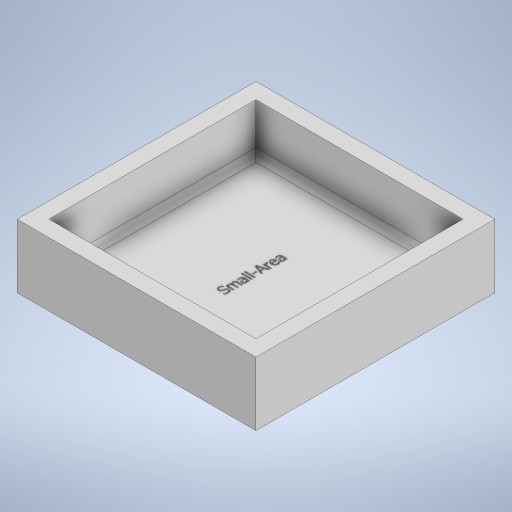
# Autodesk Inventor part: Small_Tower
Saved by Autodesk Inventor 2024.3 (Build 283343000, 343)
## iProperties
Created: 2024-08-06
Part Number: Small_Tower
Material: Generic
Document SubType Name: Modeling
Designer: lordk
Density: 1 g/cm^3
Appearance: Default
Author: lordk
Autodesk Inventor part; units mm, degrees
ref_plane "YZ Plane" through (0, 0, 0) normal (1, 0, 0) x (0, 1, 0)
ref_plane "XZ Plane" through (0, 0, 0) normal (0, 1, 0) x (-1, 0, 0)
ref_plane "XY Plane" through (0, 0, 0) normal (0, 0, 1) x (1, 0, 0)
sketch "Sketch1" plane through (0, 0, 0) normal (0, 1, 0) x (-1, 0, 0)
  line L0 (-37.5, 37.5) -> (37.5, 37.5)
  line L1 (37.5, 37.5) -> (37.5, -37.5)
  line L2 (37.5, -37.5) -> (-37.5, -37.5)
  line L3 (-37.5, -37.5) -> (-37.5, 37.5)
  line L4 (-37.5, 37.5) -> (37.5, -37.5) construction
  line L5 (37.5, 37.5) -> (-37.5, -37.5) construction
  point P0 (0, 0)
  dimension "d0" = 75
  dimension "d1" = 75
  constraints: 12 end point, 2 midpoint, 2 parallel, 1 horizontal, 1 perpendicular
  measures "d0" distance of L1.end L2.end
  measures "d1" distance of L0.end L1.end
extrude "Extrusion1" add sketch "Sketch1" along normal blind 20
sketch "Sketch2" plane through (0, 20, 0) normal (0, 1, 0) x (1, 0, 0)
  point P0 (0, 0)
shell "Shell1" thickness 5 removed faces 1 at (12.5, 20, 12.5)
fillet "Fillet1" radius 2 4 edges at (-32.5, 5, 0) (0, 5, -32.5) (0, 5, 32.5) (32.5, 5, 0)
sketch "Sketch3" plane through (-30.5, 5, -30.5) normal (0, 1, 0) x (1, 0, 0)
  line L0 (28, -41) -> (28, -20) construction
  line L1 (28, -20) -> (31, -20) construction
  line L2 (31, -20) -> (31, -41) construction
  line L3 (31, -41) -> (28, -41) construction
  line L4 (-2, 2) -> (-2, -63) projected
  line L5 (0, 0) -> (61, 0) projected
  line L6 (61, -61) -> (0, -61) projected
  line L7 (61, 0) -> (61, -61) projected
  spline S0 degree 2 poles (31.2382, -39.8416) (31.2382, -40.1725) (31.0999, -40.6369) (31.0011, -40.8419) knots 0 0 0 1 2 2 2
  line L8 (31.0011, -40.8419) -> (30.4922, -40.8419)
  line L9 (30.4922, -40.8419) -> (30.4922, -40.8123)
  spline S1 degree 2 poles (30.4922, -40.8123) (30.68, -40.6122) (30.8874, -40.1059) (30.8874, -39.8712) knots 0 0 0 1 2 2 2
  spline S2 degree 2 poles (30.8874, -39.8712) (30.8874, -39.5353) (30.6083, -39.1919) (30.3786, -39.1919) knots 0 0 0 1 2 2 2
  spline S3 degree 2 poles (30.3786, -39.1919) (30.1958, -39.1919) (29.9686, -39.3723) (29.9118, -39.5674) knots 0 0 0 1 2 2 2
  spline S4 degree 2 poles (29.9118, -39.5674) (29.8723, -39.7082) (29.8179, -39.9428) (29.7735, -40.1182) knots 0 0 0 1 2 2 2
  spline S5 degree 2 poles (29.7735, -40.1182) (29.7315, -40.2763) (29.6055, -40.5258) (29.5042, -40.6221) knots 0 0 0 1 2 2 2
  spline S6 degree 2 poles (29.5042, -40.6221) (29.403, -40.7159) (29.1313, -40.8197) (28.9534, -40.8197) knots 0 0 0 1 2 2 2
  spline S7 degree 2 poles (28.9534, -40.8197) (28.5829, -40.8197) (28.0815, -40.2417) (28.0815, -39.7946) knots 0 0 0 1 2 2 2
  spline S8 degree 2 poles (28.0815, -39.7946) (28.0815, -39.5378) (28.1828, -39.0833) (28.2791, -38.8881) knots 0 0 0 1 2 2 2
  line L10 (28.2791, -38.8881) -> (28.7632, -38.8881)
  line L11 (28.7632, -38.8881) -> (28.7632, -38.9178)
  spline S9 degree 2 poles (28.7632, -38.9178) (28.6299, -39.0635) (28.4323, -39.518) (28.4323, -39.7675) knots 0 0 0 1 2 2 2
  spline S10 degree 2 poles (28.4323, -39.7675) (28.4323, -40.049) (28.6965, -40.3973) (28.9114, -40.3973) knots 0 0 0 1 2 2 2
  spline S11 degree 2 poles (28.9114, -40.3973) (29.1041, -40.3973) (29.3338, -40.1923) (29.3857, -39.9996) knots 0 0 0 1 2 2 2
  spline S12 degree 2 poles (29.3857, -39.9996) (29.4203, -39.8712) (29.5092, -39.4982) (29.5462, -39.3747) knots 0 0 0 1 2 2 2
  spline S13 degree 2 poles (29.5462, -39.3747) (29.6426, -39.061) (30.0304, -38.7696) (30.3144, -38.7696) knots 0 0 0 1 2 2 2
  spline S14 degree 2 poles (30.3144, -38.7696) (30.4947, -38.7696) (30.8405, -38.9153) (30.9615, -39.0462) knots 0 0 0 1 2 2 2
  spline S15 degree 2 poles (30.9615, -39.0462) (31.0949, -39.1919) (31.2382, -39.5625) (31.2382, -39.8416) knots 0 0 0 1 2 2 2
  line L12 (31.1839, -35.7932) -> (29.8599, -35.7932)
  spline S16 degree 2 poles (29.8599, -35.7932) (29.7018, -35.7932) (29.4326, -35.8179) (29.3585, -35.8574) knots 0 0 0 1 2 2 2
  spline S17 degree 2 poles (29.3585, -35.8574) (29.277, -35.8969) (29.198, -36.0476) (29.198, -36.1785) knots 0 0 0 1 2 2 2
  spline S18 degree 2 poles (29.198, -36.1785) (29.198, -36.2971) (29.3437, -36.5688) (29.482, -36.7121) knots 0 0 0 1 2 2 2
  spline S19 degree 2 poles (29.482, -36.7121) (29.5166, -36.7096) (29.6129, -36.7046) (29.6771, -36.7046) knots 0 0 0 1 2 2 2
  line L13 (29.6771, -36.7046) -> (31.1839, -36.7046)
  line L14 (31.1839, -36.7046) -> (31.1839, -37.09)
  line L15 (31.1839, -37.09) -> (29.8599, -37.09)
  spline S20 degree 2 poles (29.8599, -37.09) (29.7018, -37.09) (29.4326, -37.1147) (29.3585, -37.1542) knots 0 0 0 1 2 2 2
  spline S21 degree 2 poles (29.3585, -37.1542) (29.277, -37.1937) (29.198, -37.3444) (29.198, -37.4753) knots 0 0 0 1 2 2 2
  spline S22 degree 2 poles (29.198, -37.4753) (29.198, -37.5988) (29.3536, -37.873) (29.4746, -38.0014) knots 0 0 0 1 2 2 2
  line L16 (29.4746, -38.0014) -> (31.1839, -38.0014)
  line L17 (31.1839, -38.0014) -> (31.1839, -38.3867)
  line L18 (31.1839, -38.3867) -> (28.8966, -38.3867)
  line L19 (28.8966, -38.3867) -> (28.8966, -38.0014)
  line L20 (28.8966, -38.0014) -> (29.1486, -38.0014)
  spline S23 degree 2 poles (29.1486, -38.0014) (28.9979, -37.8507) (28.8324, -37.5543) (28.8324, -37.3765) knots 0 0 0 1 2 2 2
  spline S24 degree 2 poles (28.8324, -37.3765) (28.8324, -37.1739) (29.0176, -36.8603) (29.2276, -36.7787) knots 0 0 0 1 2 2 2
  spline S25 degree 2 poles (29.2276, -36.7787) (29.0325, -36.6034) (28.8324, -36.2724) (28.8324, -36.0797) knots 0 0 0 1 2 2 2
  spline S26 degree 2 poles (28.8324, -36.0797) (28.8324, -35.9315) (28.9238, -35.6895) (29.0275, -35.6005) knots 0 0 0 1 2 2 2
  spline S27 degree 2 poles (29.0275, -35.6005) (29.1313, -35.5092) (29.4425, -35.4079) (29.6771, -35.4079) knots 0 0 0 1 2 2 2
  line L21 (29.6771, -35.4079) -> (31.1839, -35.4079)
  line L22 (31.1839, -35.4079) -> (31.1839, -35.7932)
  spline S28 degree 2 poles (30.9418, -33.5924) (30.9764, -33.6394) (31.0999, -33.7974) (31.1369, -33.8715) knots 0 0 0 1 2 2 2
  spline S29 degree 2 poles (31.1369, -33.8715) (31.1913, -33.9728) (31.2481, -34.163) (31.2481, -34.3359) knots 0 0 0 1 2 2 2
  spline S30 degree 2 poles (31.2481, -34.3359) (31.2481, -34.4767) (31.1419, -34.7311) (31.0455, -34.8274) knots 0 0 0 1 2 2 2
  spline S31 degree 2 poles (31.0455, -34.8274) (30.9517, -34.9188) (30.675, -35.03) (30.5219, -35.03) knots 0 0 0 1 2 2 2
  spline S32 degree 2 poles (30.5219, -35.03) (30.2848, -35.03) (29.9488, -34.8299) (29.8525, -34.6125) knots 0 0 0 1 2 2 2
  spline S33 degree 2 poles (29.8525, -34.6125) (29.7636, -34.4199) (29.6969, -33.8962) (29.6796, -33.5924) knots 0 0 0 1 2 2 2
  line L23 (29.6796, -33.5924) -> (29.6055, -33.5924)
  spline S34 degree 2 poles (29.6055, -33.5924) (29.4721, -33.5924) (29.3066, -33.6739) (29.2597, -33.748) knots 0 0 0 1 2 2 2
  spline S35 degree 2 poles (29.2597, -33.748) (29.2128, -33.8221) (29.1831, -34.0346) (29.1831, -34.1482) knots 0 0 0 1 2 2 2
  spline S36 degree 2 poles (29.1831, -34.1482) (29.1831, -34.2816) (29.2622, -34.6422) (29.3387, -34.8225) knots 0 0 0 1 2 2 2
  line L24 (29.3387, -34.8225) -> (29.3387, -34.8447)
  line L25 (29.3387, -34.8447) -> (28.946, -34.8447)
  spline S37 degree 2 poles (28.946, -34.8447) (28.9164, -34.7385) (28.8423, -34.3408) (28.8423, -34.1457) knots 0 0 0 1 2 2 2
  spline S38 degree 2 poles (28.8423, -34.1457) (28.8423, -33.9086) (28.9164, -33.585) (29.0127, -33.4566) knots 0 0 0 1 2 2 2
  spline S39 degree 2 poles (29.0127, -33.4566) (29.1066, -33.3306) (29.4054, -33.2071) (29.6203, -33.2071) knots 0 0 0 1 2 2 2
  line L26 (29.6203, -33.2071) -> (31.1839, -33.2071)
  line L27 (31.1839, -33.2071) -> (31.1839, -33.5924)
  line L28 (31.1839, -33.5924) -> (30.9418, -33.5924)
  line L29 (30.6207, -33.5924) -> (29.9859, -33.5924)
  spline S40 degree 2 poles (29.9859, -33.5924) (29.9982, -33.7307) (30.0402, -34.1482) (30.0798, -34.2791) knots 0 0 0 1 2 2 2
  spline S41 degree 2 poles (30.0798, -34.2791) (30.1267, -34.4322) (30.3218, -34.6323) (30.4947, -34.6323) knots 0 0 0 1 2 2 2
  spline S42 degree 2 poles (30.4947, -34.6323) (30.6923, -34.6323) (30.8924, -34.41) (30.8924, -34.1976) knots 0 0 0 1 2 2 2
  spline S43 degree 2 poles (30.8924, -34.1976) (30.8924, -34.0173) (30.7368, -33.7209) (30.6207, -33.5924) knots 0 0 0 1 2 2 2
  line L30 (31.1839, -32.2734) -> (31.1839, -32.6588)
  line L31 (31.1839, -32.6588) -> (28, -32.6588)
  line L32 (28, -32.6588) -> (28, -32.2734)
  line L33 (28, -32.2734) -> (31.1839, -32.2734)
  line L34 (31.1839, -31.3151) -> (31.1839, -31.7004)
  line L35 (31.1839, -31.7004) -> (28, -31.7004)
  line L36 (28, -31.7004) -> (28, -31.3151)
  line L37 (28, -31.3151) -> (31.1839, -31.3151)
  line L38 (30.0353, -29.6898) -> (30.0353, -30.8433)
  line L39 (30.0353, -30.8433) -> (29.6648, -30.8433)
  line L40 (29.6648, -30.8433) -> (29.6648, -29.6898)
  line L41 (29.6648, -29.6898) -> (30.0353, -29.6898)
  line L42 (31.1839, -29.5268) -> (28.1359, -28.4992)
  line L43 (28.1359, -28.4992) -> (28.1359, -28.0003)
  line L44 (28.1359, -28.0003) -> (31.1839, -26.9728)
  line L45 (31.1839, -26.9728) -> (31.1839, -27.4001)
  line L46 (31.1839, -27.4001) -> (30.3317, -27.6767)
  line L47 (30.3317, -27.6767) -> (30.3317, -28.8401)
  line L48 (30.3317, -28.8401) -> (31.1839, -29.1168)
  line L49 (31.1839, -29.1168) -> (31.1839, -29.5268)
  line L50 (29.9859, -27.7879) -> (28.5508, -28.2597)
  line L51 (28.5508, -28.2597) -> (29.9859, -28.729)
  line L52 (29.9859, -28.729) -> (29.9859, -27.7879)
  line L53 (29.3091, -25.5006) -> (29.3091, -25.5204)
  spline S44 degree 2 poles (29.3091, -25.5204) (29.2968, -25.5649) (29.2918, -25.6612) (29.2918, -25.7279) knots 0 0 0 1 2 2 2
  spline S45 degree 2 poles (29.2918, -25.7279) (29.2918, -25.8835) (29.4277, -26.1898) (29.5611, -26.3281) knots 0 0 0 1 2 2 2
  line L54 (29.5611, -26.3281) -> (31.1839, -26.3281)
  line L55 (31.1839, -26.3281) -> (31.1839, -26.7134)
  line L56 (31.1839, -26.7134) -> (28.8966, -26.7134)
  line L57 (28.8966, -26.7134) -> (28.8966, -26.3281)
  line L58 (28.8966, -26.3281) -> (29.2375, -26.3281)
  spline S46 degree 2 poles (29.2375, -26.3281) (29.0498, -26.1182) (28.8966, -25.8045) (28.8966, -25.6563) knots 0 0 0 1 2 2 2
  spline S47 degree 2 poles (28.8966, -25.6563) (28.8966, -25.597) (28.9016, -25.5377) (28.909, -25.5006) knots 0 0 0 1 2 2 2
  line L59 (28.909, -25.5006) -> (29.3091, -25.5006)
  spline S48 degree 2 poles (31.2357, -24.2088) (31.2357, -24.7572) (30.6207, -25.3599) (30.0526, -25.3599) knots 0 0 0 1 2 2 2
  spline S49 degree 2 poles (30.0526, -25.3599) (29.4944, -25.3599) (28.8324, -24.7745) (28.8324, -24.3027) knots 0 0 0 1 2 2 2
  spline S50 degree 2 poles (28.8324, -24.3027) (28.8324, -24.0903) (28.9559, -23.7618) (29.0868, -23.6407) knots 0 0 0 1 2 2 2
  spline S51 degree 2 poles (29.0868, -23.6407) (29.2177, -23.5172) (29.5956, -23.3863) (29.8698, -23.3863) knots 0 0 0 1 2 2 2
  line L60 (29.8698, -23.3863) -> (30.0798, -23.3863)
  line L61 (30.0798, -23.3863) -> (30.0798, -24.9696)
  spline S52 degree 2 poles (30.0798, -24.9696) (30.4774, -24.9696) (30.8998, -24.5695) (30.8998, -24.2138) knots 0 0 0 1 2 2 2
  spline S53 degree 2 poles (30.8998, -24.2138) (30.8998, -24.0878) (30.843, -23.8433) (30.7985, -23.7445) knots 0 0 0 1 2 2 2
  spline S54 degree 2 poles (30.7985, -23.7445) (30.7491, -23.6407) (30.6627, -23.4975) (30.6232, -23.4505) knots 0 0 0 1 2 2 2
  line L62 (30.6232, -23.4505) -> (30.6232, -23.4283)
  line L63 (30.6232, -23.4283) -> (31.0431, -23.4283)
  spline S55 degree 2 poles (31.0431, -23.4283) (31.0702, -23.495) (31.1493, -23.6975) (31.1715, -23.7766) knots 0 0 0 1 2 2 2
  spline S56 degree 2 poles (31.1715, -23.7766) (31.2036, -23.8877) (31.2357, -24.0705) (31.2357, -24.2088) knots 0 0 0 1 2 2 2
  spline S57 degree 2 poles (29.7858, -23.7618) (29.6302, -23.7667) (29.403, -23.8309) (29.3264, -23.8927) knots 0 0 0 1 2 2 2
  spline S58 degree 2 poles (29.3264, -23.8927) (29.2399, -23.9594) (29.1486, -24.1693) (29.1486, -24.3249) knots 0 0 0 1 2 2 2
  spline S59 degree 2 poles (29.1486, -24.3249) (29.1486, -24.4781) (29.2399, -24.693) (29.3289, -24.7819) knots 0 0 0 1 2 2 2
  spline S60 degree 2 poles (29.3289, -24.7819) (29.4203, -24.8683) (29.6401, -24.9572) (29.7858, -24.9696) knots 0 0 0 1 2 2 2
  line L64 (29.7858, -24.9696) -> (29.7858, -23.7618)
  spline S61 degree 2 poles (30.9418, -21.7215) (30.9764, -21.7685) (31.0999, -21.9265) (31.1369, -22.0006) knots 0 0 0 1 2 2 2
  spline S62 degree 2 poles (31.1369, -22.0006) (31.1913, -22.1019) (31.2481, -22.2921) (31.2481, -22.465) knots 0 0 0 1 2 2 2
  spline S63 degree 2 poles (31.2481, -22.465) (31.2481, -22.6058) (31.1419, -22.8602) (31.0455, -22.9565) knots 0 0 0 1 2 2 2
  spline S64 degree 2 poles (31.0455, -22.9565) (30.9517, -23.0479) (30.675, -23.1591) (30.5219, -23.1591) knots 0 0 0 1 2 2 2
  spline S65 degree 2 poles (30.5219, -23.1591) (30.2848, -23.1591) (29.9488, -22.959) (29.8525, -22.7416) knots 0 0 0 1 2 2 2
  spline S66 degree 2 poles (29.8525, -22.7416) (29.7636, -22.549) (29.6969, -22.0253) (29.6796, -21.7215) knots 0 0 0 1 2 2 2
  line L65 (29.6796, -21.7215) -> (29.6055, -21.7215)
  spline S67 degree 2 poles (29.6055, -21.7215) (29.4721, -21.7215) (29.3066, -21.803) (29.2597, -21.8771) knots 0 0 0 1 2 2 2
  spline S68 degree 2 poles (29.2597, -21.8771) (29.2128, -21.9512) (29.1831, -22.1637) (29.1831, -22.2773) knots 0 0 0 1 2 2 2
  spline S69 degree 2 poles (29.1831, -22.2773) (29.1831, -22.4107) (29.2622, -22.7713) (29.3387, -22.9516) knots 0 0 0 1 2 2 2
  line L66 (29.3387, -22.9516) -> (29.3387, -22.9738)
  line L67 (29.3387, -22.9738) -> (28.946, -22.9738)
  spline S70 degree 2 poles (28.946, -22.9738) (28.9164, -22.8676) (28.8423, -22.4699) (28.8423, -22.2748) knots 0 0 0 1 2 2 2
  spline S71 degree 2 poles (28.8423, -22.2748) (28.8423, -22.0377) (28.9164, -21.7141) (29.0127, -21.5857) knots 0 0 0 1 2 2 2
  spline S72 degree 2 poles (29.0127, -21.5857) (29.1066, -21.4597) (29.4054, -21.3362) (29.6203, -21.3362) knots 0 0 0 1 2 2 2
  line L68 (29.6203, -21.3362) -> (31.1839, -21.3362)
  line L69 (31.1839, -21.3362) -> (31.1839, -21.7215)
  line L70 (31.1839, -21.7215) -> (30.9418, -21.7215)
  line L71 (30.6207, -21.7215) -> (29.9859, -21.7215)
  spline S73 degree 2 poles (29.9859, -21.7215) (29.9982, -21.8598) (30.0402, -22.2773) (30.0798, -22.4082) knots 0 0 0 1 2 2 2
  spline S74 degree 2 poles (30.0798, -22.4082) (30.1267, -22.5613) (30.3218, -22.7614) (30.4947, -22.7614) knots 0 0 0 1 2 2 2
  spline S75 degree 2 poles (30.4947, -22.7614) (30.6923, -22.7614) (30.8924, -22.5391) (30.8924, -22.3267) knots 0 0 0 1 2 2 2
  spline S76 degree 2 poles (30.8924, -22.3267) (30.8924, -22.1464) (30.7368, -21.85) (30.6207, -21.7215) knots 0 0 0 1 2 2 2
  point P0 (30.5, -30.5)
  point P1 (29.5, -20)
  point P2 (29.5, -41)
  dimension "d6" = 30
  dimension "d7" = 20
  dimension "d8" = 20
  dimension "d9" = 30
  constraints: 2 midpoint, 2 other
  measures "d6" distance between parallel lines of L4 L0
  measures "d7" distance from line of L5 point (29.5, -20)
  measures "d8" distance from line of L6 point (29.5, -41)
  measures "d9" distance between parallel lines of L7 L2
extrude "Extrusion2" cut sketch "Sketch3" against normal blind 1
body "Solid1"
